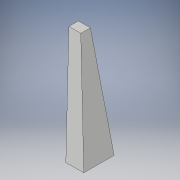
# Autodesk Inventor part: slide upright
Saved by Autodesk Inventor 2019 (Build 230136000, 136)
## iProperties
Created: 2020-01-04
Part Number: slide upright
Material: Generic
Document SubType Name: Modeling
Designer: User
Density: 1 g/cm^3
Appearance: Default
Author: User
Autodesk Inventor part; units mm, degrees
ref_plane "YZ Plane" through (0, 0, 0) normal (1, 0, 0) x (0, 1, 0)
ref_plane "XZ Plane" through (0, 0, 0) normal (0, 1, 0) x (-1, 0, 0)
ref_plane "XY Plane" through (0, 0, 0) normal (0, 0, 1) x (1, 0, 0)
sketch "Sketch1" plane through (0, 0, 0) normal (1, 0, 0) x (0, 1, 0)
  line L0 (0, 0) -> (254, 0)
  line L1 (254, 0) -> (254, -20.32)
  line L2 (254, -20.32) -> (6.4008, -63.5)
  line L3 (6.4008, -63.5) -> (0, -63.5)
  line L4 (0, -63.5) -> (0, 0)
  dimension "d0" = 254
  dimension "d1" = 20.32
  dimension "d2" = 6.4008
  dimension "d3" = 63.5
  constraints: 10 end point, 2 perpendicular, 1 horizontal, 1 parallel
  measures "d0" distance of L0.start L0.end
  measures "d1" distance of L0.end L1.end
  measures "d2" distance of L2.end L3.end
  measures "d3" distance of L3.end L0.start
extrude "Extrusion1" add sketch "Sketch1" along normal blind 20.701
sketch "Sketch2" plane through (0, 0, -63.5) normal (0, 0, -1) x (-1, 0, 0)
  line L0 (-20.701, 238.8682) -> (0, 238.8682)
  line L1 (0, 238.8682) -> (0, 17.78)
  line L2 (0, 17.78) -> (-20.701, 17.78)
  line L3 (-20.701, 17.78) -> (-20.701, 238.8682)
  line L4 (0, 254) -> (0, 6.4008) projected
  line L5 (0, 0) -> (-20.701, 0) projected
  dimension "d6" = 20.701
  dimension "d7" = 0
  dimension "d8" = 17.78
  constraints: 8 end point, 2 parallel, 1 horizontal, 1 perpendicular
  measures "d6" distance of L0.start L0.end
  measures "d7" distance between parallel lines of L4 L1
  measures "d8" distance between parallel lines of L5 L2
sketch "Sketch3" plane through (0, 0, 0) normal (0, 0, 1) x (1, 0, 0)
  line L0 (0, 254) -> (20.701, 254) projected
  line L1 (20.701, 254) -> (23.0505, 254)
  line L2 (23.0505, 254) -> (29.4005, 0)
  line L3 (29.4005, 0) -> (-8.6995, 0)
  line L4 (-8.6995, 0) -> (-2.3495, 254)
  line L5 (-2.3495, 254) -> (0, 254)
  line L6 (20.701, 254) -> (20.701, 0) projected
  point P0 (0, 0)
  dimension "d10" = 25.4
  dimension "d11" = 38.1
  dimension "d12" = 2.3495
  dimension "d13" = 254
  dimension "d14" = 8.6995
  constraints: 10 end point, 1 collinear, 1 horizontal, 1 parallel, 1 point on line
  measures "d10" distance of L1.end L4.end
  measures "d11" distance of L2.end L3.end
  measures "d12" distance of L4.end L0.start
  measures "d13" vertical distance of L3.end L4.end
  measures "d14" distance from line of L2.end L6
extrude "Extrusion2" add sketch "Sketch3" against normal up to surface surface through (0, 6.4008, -63.5) normal (0, 0.1718018, -0.9851315)
extrude "Extrusion3" cut sketch "Sketch2" against normal up to surface (43.18 mm away)
body "Solid1"
